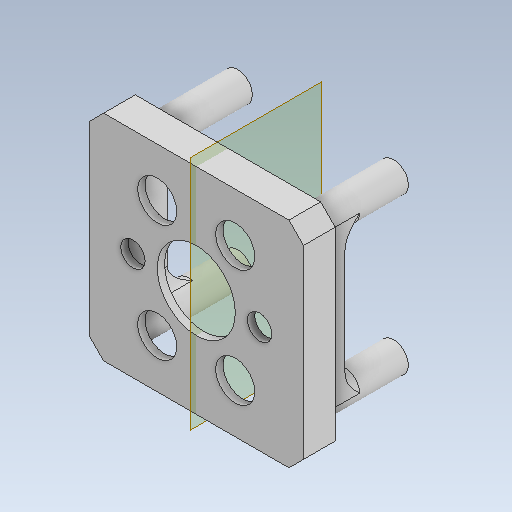
# Autodesk Inventor part: ext_shell_top
Saved by Autodesk Inventor 2020 (Build 240168000, 168)
## iProperties
Created: 2022-06-18
Part Number: ext_shell_top
Material: Generic
Document SubType Name: Modeling
Designer: Shuang Peng
Density: 1 g/cm^3
Appearance: Default
Author: Shuang Peng
Autodesk Inventor part; units mm, degrees
ref_plane "YZ Plane" through (0, 0, 0) normal (1, 0, 0) x (0, 1, 0)
ref_plane "XZ Plane" through (0, 0, 0) normal (0, 1, 0) x (-1, 0, 0)
ref_plane "XY Plane" through (0, 0, 0) normal (0, 0, 1) x (1, 0, 0)
sketch "Sketch1" plane through (0, 0, 0) normal (0, 0, 1) x (1, 0, 0)
  circle A0 centre (-16, 16) radius 1 projected
  circle A1 centre (-16, -16) radius 1 projected
  circle A2 centre (16, -16) radius 1 projected
  circle A3 centre (16, 16) radius 1 projected
  circle A4 centre (-16, 16) radius 1.2
  circle A5 centre (-16, -16) radius 1.2
  circle A6 centre (16, 16) radius 1.2
  circle A7 centre (16, -16) radius 1.2
  circle A8 centre (-16, 16) radius 3
  circle A9 centre (16, 16) radius 3
  circle A10 centre (16, -16) radius 3
  circle A11 centre (-16, -16) radius 3
  point P0 (0, 0)
  dimension "d0" = 2.4
  dimension "d1" = 2.4
  dimension "d2" = 2.4
  dimension "d3" = 2.4
  dimension "d4" = 6
  dimension "d5" = 6
  dimension "d6" = 6
  dimension "d7" = 6
  constraints: 8 centre point, 8 coincident
  measures "d0" diameter of A4
  measures "d1" diameter of A5
  measures "d2" diameter of A6
  measures "d3" diameter of A7
  measures "d4" diameter of A8
  measures "d5" diameter of A9
  measures "d6" diameter of A10
  measures "d7" diameter of A11
extrude "Extrusion1" add sketch "Sketch1" along normal blind 23 contours A8 | A9 | A10 | A11
sketch "Sketch2" plane through (-16, -16, 23) normal (0, 0, 1) x (1, 0, 0)
  line L0 (38, -6) -> (-6, -6)
  line L1 (-6, -6) -> (-6, 38)
  line L2 (-6, 38) -> (38, 38)
  line L3 (38, 38) -> (38, -6)
  line L4 (38, -6) -> (-6, 38) construction
  line L5 (-6, -6) -> (38, 38) construction
  point P0 (16, 16)
  dimension "d10" = 44
  dimension "d11" = 44
  constraints: 12 end point, 2 midpoint, 2 parallel, 1 horizontal, 1 perpendicular
  measures "d10" distance of L0.start L0.end
  measures "d11" distance of L0.end L1.end
extrude "Extrusion2" add sketch "Sketch2" along normal blind 1.5
sketch "Sketch3" plane through (-16, -16, 23) normal (0, 0, -1) x (-1, 0, 0)
  line L0 (3, 33) -> (3, -1) projected
  circle A0 centre (0, 32) radius 3 projected
  circle A1 centre (0, 0) radius 3 projected
  line L1 (1.5, 29.4019) -> (1.5, 2.5981)
  point P0 (-16, 16)
  point P1 (3, 0)
  point P2 (3, 32)
  dimension "d14" = 1.5
  constraints: 2 end point, 1 vertical, 4 other
  measures "d14" distance between parallel lines of L0 L1
extrude "Extrusion3" add sketch "Sketch3" along normal blind 10 contours L0 A1 L1 A0
ref_plane "Work Plane1" through (0, -22, 23) normal (-1, 0, 0) x (0, 0, 1)
mirror "Mirror1" about plane through (0, -22, 23) normal (-1, 0, 0) of "Extrusion3"
fillet "Fillet1" radius 3 4 edges at (17.5, 13.4019, 18) (17.5, -13.4019, 18) (-17.5, -13.4019, 18) (-17.5, 13.4019, 18)
fillet "Fillet2" radius 1 14 edges at (14.1629, 18.3717, 23) (16.8717, 12.0276, 23) (17.5, 0, 23) (16.8717, -12.0276, 23) (14.1629, -18.3717, 23) (19, 0, 23) (-13.6283, -14.1629, 23) (-16, -19, 23) (-16.8717, -12.0276, 23) (-17.5, 0, 23) (-16.8717, 12.0276, 23) (-16, 19, 23) (-13.6283, 14.1629, 23) (-19, 0, 23)
fillet "Fillet3" radius 3 8 edges at (16.4051, 13.0275, 13) (18.5981, 14.5, 13) (16.4051, -13.0275, 13) (18.5981, -14.5, 13) (-16.4051, -13.0275, 13) (-18.5981, -14.5, 13) (-16.4051, 13.0275, 13) (-18.5981, 14.5, 13)
chamfer "Chamfer1" distance 1.3 angle 70 1 edges at (14.8, 16, 0) measured on face at (14.3, 16, 0)
chamfer "Chamfer2" distance 1.3 angle 70 1 edges at (14.8, -16, 0) measured on face at (14.3, -16, 0)
chamfer "Chamfer3" distance 1.3 angle 70 1 edges at (-17.2, -16, 0) measured on face at (-17.7, -16, 0)
chamfer "Chamfer4" distance 1.3 angle 70 1 edges at (-17.2, 16, 0) measured on face at (-17.7, 16, 0)
sketch "Sketch4" plane through (-16, -16, 23) normal (0, 0, -1) x (-1, 0, 0)
  arc A0 (-31, 28.127) -> (-36, 32) centre (-32, 32) ccw projected
  arc A1 (-31, 28.127) -> (-32.5, 26.1905) centre (-30.5, 26.1905) ccw projected
  line L0 (-32.5, 5.8095) -> (-32.5, 26.1905) projected
  arc A2 (-32.5, 5.8095) -> (-31, 3.873) centre (-30.5, 5.8095) ccw projected
  arc A3 (-36, 0) -> (-31, 3.873) centre (-32, 0) ccw projected
  line L1 (-36, 32) -> (-36, 0) projected
  line L2 (6, 38) -> (6, -6) projected
  line L3 (-38, 38) -> (6, 38) projected
  line L4 (-38, -6) -> (-38, 38) projected
  line L5 (6, -6) -> (-38, -6) projected
  arc A4 (-1, 3.873) -> (4, 0) centre (0, 0) ccw projected
  arc A5 (-1, 3.873) -> (0.5, 5.8095) centre (-1.5, 5.8095) ccw projected
  line L6 (0.5, 26.1905) -> (0.5, 5.8095) projected
  arc A6 (0.5, 26.1905) -> (-1, 28.127) centre (-1.5, 26.1905) ccw projected
  arc A7 (4, 32) -> (-1, 28.127) centre (0, 32) ccw projected
  line L7 (4, 0) -> (4, 32) projected
  line L8 (-37, -5) -> (-37, 37)
  line L9 (-37, 37) -> (5, 37)
  line L10 (5, 37) -> (5, -5)
  line L11 (5, -5) -> (-37, -5)
  line L12 (-37, -5) -> (5, 37) construction
  line L13 (-37, 37) -> (5, -5) construction
  point P0 (-16, 16)
  dimension "d32" = 1
  dimension "d33" = 1
  constraints: 12 end point, 2 midpoint, 2 parallel, 1 perpendicular, 1 vertical
  measures "d32" distance between parallel lines of L3 L9
  measures "d33" distance between parallel lines of L2 L10
extrude "Extrusion4" add sketch "Sketch4" along normal blind 5 contours L2 L5 L4 L3
chamfer "Chamfer5" distance 3 angle 45 4 edges at (21, -21, 20.5) (21, 21, 20.5) (-21, 21, 20.5) (-21, -21, 20.5)
chamfer "Chamfer6" distance 3 angle 45 4 edges at (-22, -22, 21.25) (-22, 22, 21.25) (22, 22, 21.25) (22, -22, 21.25)
sketch "Sketch5" plane through (-16, -16, 23) normal (0, 0, -1) x (-1, 0, 0)
  line L0 (-38, 35) -> (-38, -3) projected
  line L1 (6, -3) -> (6, 35) projected
  arc A0 (1.5, 26.1905) -> (3, 26.8038) centre (0, 32) ccw projected
  line L2 (1.5, 26.1905) -> (1.5, 5.8095) projected
  arc A1 (3, 5.1962) -> (1.5, 5.8095) centre (0, 0) ccw projected
  line L3 (3, 5.1962) -> (3, 26.8038) projected
  arc A2 (-33.5, 5.8095) -> (-35, 5.1962) centre (-32, 0) ccw projected
  line L4 (-33.5, 26.1905) -> (-33.5, 5.8095) projected
  arc A3 (-35, 26.8038) -> (-33.5, 26.1905) centre (-32, 32) ccw projected
  line L5 (-35, 5.1962) -> (-35, 26.8038) projected
  line L6 (-41, 14.5) -> (-41, 17.5)
  line L7 (-41, 17.5) -> (9, 17.5)
  line L8 (9, 17.5) -> (9, 14.5)
  line L9 (9, 14.5) -> (-41, 14.5)
  line L10 (-41, 14.5) -> (9, 17.5) construction
  line L11 (-41, 17.5) -> (9, 14.5) construction
  point P0 (-16, 16)
  point P1 (3, 14.5)
  point P2 (6, 14.5)
  point P3 (6, 17.5)
  point P4 (3, 17.5)
  point P5 (-38, 14.5)
  point P6 (-35, 14.5)
  point P7 (-35, 17.5)
  point P8 (-38, 17.5)
  dimension "d42" = 3
  dimension "d43" = 50
  constraints: 12 end point, 2 midpoint, 2 parallel, 1 perpendicular, 1 vertical
  measures "d42" distance of L6.start L6.end
  measures "d43" distance of L6.end L7.end
extrude "Extrusion5" add sketch "Sketch5" along normal blind 5 contours L7 L5 L9 L0 | L7 L1 L9 L3
fillet "Fillet4" radius 0.5 16 edges at (-19.2929, -1.5, 22.7071) (-20.5, -1.5, 23) (-19, -1.5, 20) (-19.2929, 1.5, 22.7071) (-20.5, 1.5, 23) (-19, 1.5, 20) (-21, 1.5, 20.5) (-21, -1.5, 20.5) (19.2929, -1.5, 22.7071) (20.5, -1.5, 23) (19, -1.5, 20) (19, 1.5, 20) (20.5, 1.5, 23) (19.2929, 1.5, 22.7071) (21, 1.5, 20.5) (21, -1.5, 20.5)
fillet "Fillet5" radius 1 6 edges at (19, -1.75, 18) (19, 0, 18) (19, 1.75, 18) (-19, -1.75, 18) (-19, 0, 18) (-19, 1.75, 18)
fillet "Fillet6" radius 1 14 edges at (-19.5, 19.5, 23) (0, 21, 23) (19.5, 19.5, 23) (0, -21, 23) (-19.5, -19.5, 23) (19.5, -19.5, 23) (-18, -21, 20.5) (18, -21, 20.5) (21, -18, 20.5) (21, 18, 20.5) (18, 21, 20.5) (-18, 21, 20.5) (-21, 18, 20.5) (-21, -18, 20.5)
sketch "Sketch8" plane through (-16, -16, 23) normal (0, 0, -1) x (-1, 0, 0)
  circle A0 centre (-16, 16) radius 8
  line L0 (-16, 16) -> (-16, 28)
  line L1 (-16, 28) -> (-24, 28)
  circle A1 centre (-24, 28) radius 4
  line L2 (-16, 16) -> (-8, 16)
  circle A2 centre (-24, 4) radius 4
  line L3 (-16, 16) -> (-29, 16)
  circle A3 centre (-29, 16) radius 2.5
  circle A4 centre (-8, 28) radius 4
  circle A5 centre (-8, 4) radius 4
  circle A6 centre (-3, 16) radius 2.5
  dimension "d73" = 16
  dimension "d74" = 12
  dimension "d75" = 8
  dimension "d76" = 8
  dimension "d77" = 13
  dimension "d78" = 5
  constraints: 8 end point, 6 centre point, 4 symmetric about line, 3 coincident, 2 horizontal, 1 horizontal alignment, 1 perpendicular, 1 vertical, 6 other
  measures "d74" distance of L0.start L0.end
  measures "d75" distance of L0.end L1.end
  measures "d76" diameter of A1
  measures "d77" distance of L0.start L3.end
  measures "d78" diameter of A3
extrude "Extrusion7" cut sketch "Sketch8" against normal blind 5
body "Solid1"
